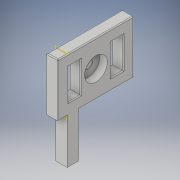
# Autodesk Inventor part: TensionerPlate
Saved by Autodesk Inventor 2017 (Build 210142000, 142)
## iProperties
Created: 2017-07-29
Part Number: TensionerPlate
Material: Generic
Document SubType Name: Modeling
Designer: User
Density: 1 g/cm^3
Appearance: Default
Author: User
Autodesk Inventor part; units mm, degrees
ref_plane "YZ Plane" through (0, 0, 0) normal (1, 0, 0) x (0, 1, 0)
ref_plane "XZ Plane" through (0, 0, 0) normal (0, 1, 0) x (-1, 0, 0)
ref_plane "XY Plane" through (0, 0, 0) normal (0, 0, 1) x (1, 0, 0)
sketch "Sketch1" plane through (0, 0, 0) normal (1, 0, 0) x (0, 1, 0)
  line L0 (22.225, 0) -> (22.225, -31.75)
  line L1 (22.225, -31.75) -> (0, -31.75)
  line L2 (0, -31.75) -> (0, 0)
  line L3 (17.5895, -4.5085) -> (4.8895, -4.5085)
  line L4 (6.35, -31.75) -> (25.4, -31.75)
  line L5 (0, 0) -> (4.7625, 0)
  line L6 (17.5895, 0) -> (22.225, 0)
  line L7 (4.6355, -22.225) -> (17.5895, -22.225)
  line L8 (17.5895, -22.225) -> (17.5895, -27.2415)
  line L9 (17.5895, -27.2415) -> (4.6355, -27.2415)
  line L10 (4.6355, -27.2415) -> (4.6355, -22.225)
  line L11 (22.225, 0) -> (0, 0)
  line L12 (17.5895, -4.5085) -> (4.6355, -4.5085)
  line L13 (4.6355, -4.5085) -> (4.6355, -9.525)
  line L14 (4.6355, -9.525) -> (17.5895, -9.525)
  line L15 (17.5895, -9.525) -> (17.5895, -4.5085)
  dimension "d8" = 12.954
  dimension "d9" = 5.0165
  dimension "d10" = 4.5085
  dimension "d11" = 4.6355
  dimension "d28" = 4.6355
  dimension "d29" = 4.5085
  dimension "d37" = 31.75
  dimension "d38" = 31.75
  dimension "d43" = 5.0165
  dimension "d48" = 12.954
  dimension "d49" = 4.6355
  constraints: 32 end point, 7 parallel, 5 horizontal, 4 perpendicular, 1 point on line
  measures "d8" distance of L8.end L9.end
  measures "d9" distance of L7.end L8.end
  measures "d10" distance between parallel lines of L1 L9
  measures "d11" distance between parallel lines of L2 L10
  measures "d28" distance between parallel lines of L8 L0
  measures "d29" distance of L6.start L3.start
  measures "d37" distance of L0.start L0.end
  measures "d38" distance of L1.end L2.end
  measures "d43" distance of L14.end L3.start
  measures "d48" distance of L13.end L14.end
  measures "d49" distance between parallel lines of L2 L13
extrude "Extrusion1" add sketch "Sketch1" along normal blind 4.7625 contours L0 L1 L2 L5 L11 L6 | L15 L14 L13 L12 L3
sketch "Sketch2" plane through (4.7625, 0, 0) normal (1, 0, 0) x (0, 0, -1)
  line L0 (22.225, 17.5895) -> (27.2415, 17.5895) projected
  line L1 (27.2415, 17.5895) -> (27.2415, 4.6355) projected
  line L2 (27.2415, 4.6355) -> (22.225, 4.6355) projected
  line L3 (22.225, 4.6355) -> (22.225, 17.5895) projected
  line L4 (0, 0) -> (31.75, 0) projected
  line L5 (31.75, 0) -> (31.75, 22.225) projected
  line L6 (31.75, 22.225) -> (0, 22.225) projected
  circle A0 centre (15.875, 11.1125) radius 4.7625
  line L7 (0, 22.225) -> (0, 0) projected
  dimension "d14" = 9.525
  dimension "d15" = 11.1125
  dimension "d39" = 22.225
  dimension "d52" = 31.75
  dimension "d53" = 15.875
  constraints: 1 centre point
  measures "d14" diameter of A0
  measures "d15" distance from line of L6 A0.centre
  measures "d39" distance of L4.end L5.end
  measures "d52" distance of L5.end L6.end
  measures "d53" distance from line of L7 A0.centre
extrude "Extrusion2" cut sketch "Sketch2" against normal blind 3.175 contours A0
extrude "Extrusion5" cut sketch "Sketch1" along normal blind 25.4 contours L15 L14 L13 L12 L3
sketch "Sketch5" plane through (4.7625, 0, 0) normal (1, 0, 0) x (0, 0, -1)
  circle A0 centre (15.875, 11.1125) radius 4.7625 projected
  point P0 (0, 0)
  constraints: 1 coincident
hole "Hole1" at (4.7625, 11.1125, -15.875) direction (-1, 0, 0) diameter 3.683 depth 14.9352 tip angle 118 thread size "10-24 UNC" class "2B" standard "ANSI Unified Screw Threads"
fillet "Fillet1" radius 0.381 26 edges at (0, 22.225, -15.875) (2.3813, 22.225, 0) (4.7625, 22.225, -15.875) (4.7625, 11.1125, -31.75) (0, 11.1125, -31.75) (4.7625, 0, -15.875) (2.3813, 0, -31.75) (4.7625, 11.1125, 0) (4.7625, 11.1125, -4.5085) (4.7625, 17.5895, -7.0167) (4.7625, 11.1125, -9.525) (4.7625, 4.6355, -7.0167) (0, 4.6355, -7.0167) (0, 11.1125, -4.5085) (2.3813, 22.225, -31.75) (4.7625, 17.5895, -24.7332) (4.7625, 11.1125, -22.225) (4.7625, 4.6355, -24.7332) (4.7625, 11.1125, -27.2415) (0, 17.5895, -24.7332) (0, 11.1125, -27.2415) (0, 11.1125, -22.225) (0, 4.6355, -24.7332) (0, 11.1125, -9.525) (0, 17.5895, -7.0167) (0, 0, -15.875)
ref_plane "Work Plane1" through (0, 0.381, -3.81) normal (0, 0, 1) x (1, 0, 0)
sketch "Sketch7" plane through (0, 0.381, -3.81) normal (0, 0, 1) x (1, 0, 0)
  line L0 (0, 21.463) -> (4.3815, 21.463) projected
  line L1 (0, 21.463) -> (0, 0) projected
  arc A0 (0, 0) -> (0.381, -0.381) centre (0.381, 0) ccw projected
  line L2 (0.381, -0.381) -> (4.3815, -0.381) projected
  line L3 (4.3815, 21.463) -> (4.3815, -0.381) projected
  line L4 (4.7625, 0) -> (4.7625, 21.463) projected
  line L5 (0, 21.463) -> (0, 0) projected
  line L6 (0, 0) -> (4.7625, 0)
  line L7 (4.7625, 0) -> (4.7625, -19.05)
  line L8 (4.7625, -19.05) -> (0, -19.05)
  line L9 (0, -19.05) -> (0, 0)
  point P0 (0, -0.381)
  dimension "d75" = 4.7625
  dimension "d76" = 19.05
  constraints: 8 end point, 2 parallel, 1 horizontal, 1 perpendicular
  measures "d75" distance of L7.end L8.end
  measures "d76" distance of L6.end L7.end
extrude "Extrusion6" add sketch "Sketch7" against normal blind 4.7625 contours L6 L3 L2 A0 | A0 L2 L3 L6 L7 L8 L9
equation "\"d28\" = d11"
equation "\"d38\" = d37"
equation "\"d15\" = 0.5 * d39"
equation "\"d53\" = 0.5 * d52"
equation "\"d32\" = 0.5 * d31"
equation "\"d31\" = 6.274854"
body "Solid1"
